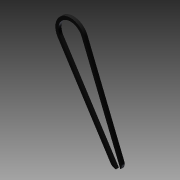
# Autodesk Inventor part: conveyor belt drive belt
Saved by Autodesk Inventor 2011 SP1 (Build 150282100, 282)
## iProperties
Created: 2012-01-20
Part Number: conveyor belt drive belt
Document SubType Name: Modeling
Designer: Christopher
Density: 1 g/cm^3
Author: Christopher
Autodesk Inventor part; units mm, degrees
ref_plane "YZ Plane" through (0, 0, 0) normal (1, 0, 0) x (0, 1, 0)
ref_plane "XZ Plane" through (0, 0, 0) normal (0, 1, 0) x (-1, 0, 0)
ref_plane "XY Plane" through (0, 0, 0) normal (0, 0, 1) x (1, 0, 0)
sketch "Sketch1" plane through (0, 0, 0) normal (0, 0, 1) x (1, 0, 0)
  circle A0 centre (95.25, 0) radius 12.7
  circle A1 centre (1.2118, 184.146) radius 31.75
  line L0 (30.6982, 195.9194) -> (107.0446, 4.7093)
  line L1 (84.5197, -6.7935) -> (-25.6139, 167.1623)
  line L2 (24.6815, 193.8637) -> (101.81, 0.6948)
  line L3 (89.702, -3.1079) -> (-25.2322, 178.4304)
  arc A2 (24.6815, 193.8637) -> (-25.2322, 178.4304) centre (0.3434, 184.146) ccw
  arc A3 (89.702, -3.1079) -> (101.81, 0.6948) centre (95.25, 0.4046) ccw
  point P0 (0, 0)
  dimension "d0" = 95.25
  dimension "d1" = 184.15
  dimension "d2" = 25.4
  dimension "d3" = 63.5
  dimension "d6" = 6.35
  dimension "d7" = 6.35
  constraints: 8 end point, 8 point on circle, 6 tangent, 4 centre point, 2 coincident, 2 horizontal alignment, 2 parallel, 1 vertical alignment
  measures "d0" distance of point (0, 0) point (95.25, 0)
  measures "d1" distance of point (1.212, 184.146) point (0, 0)
  measures "d2" diameter of A0
  measures "d3" diameter of A1
  measures "d6" distance between parallel lines of L1 L3
  measures "d7" distance between parallel lines of L0 L2
extrude "Extrusion1" add sketch "Sketch1" against normal blind 6.35
extrude "Extrusion2" cut sketch "Sketch1" against normal blind 6.35 contours L2 A3 L3 A0 | A0 L3 A1 L2 | A1 L3 A2 L2 picked at (94.1398, 3.1738) picked at (1.4272, 174.9657)
body "Solid1"
